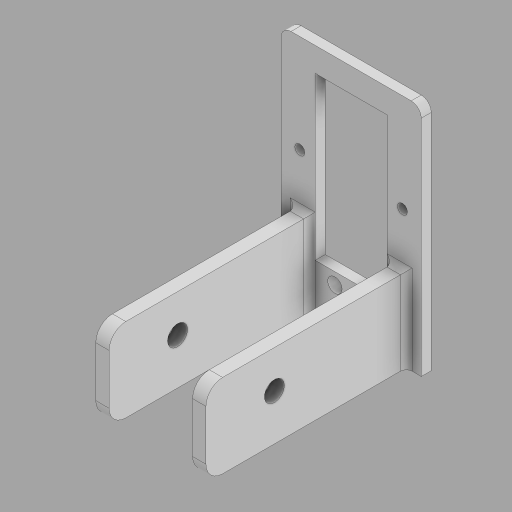
# Autodesk Inventor part: MG995_apoio
Saved by Autodesk Inventor 2023.2 (Build 272271030, 271C)
## iProperties
Created: 2023-04-15
Part Number: MG995_apoio
Material: Generic
Document SubType Name: Modeling
Designer: victo
Density: 1 g/cm^3
Appearance: Default
Author: victo
## iProperties of the stored document MG995_apoio_3DPrint.ipt
Created: 2023-07-24
Part Number: MG995_apoio_3DPrint
Material: Generic
Document SubType Name: Modeling
Designer: VICTOR
Density: 1 g/cm^3
Appearance: Default
Author: VICTOR
Autodesk Inventor part; units mm, degrees
ref_plane "YZ Plane" through (0, 0, 0) normal (1, 0, 0) x (0, 1, 0)
ref_plane "XZ Plane" through (0, 0, 0) normal (0, 1, 0) x (-1, 0, 0)
ref_plane "XY Plane" through (0, 0, 0) normal (0, 0, 1) x (1, 0, 0)
sketch "Sketch1" plane through (0, 0, 0) normal (0, 0, 1) x (1, 0, 0)
  line L0 (0, 0) -> (42, 0)
  line L1 (42, 0) -> (42, 70)
  line L2 (42, 70) -> (0, 70)
  line L3 (0, 70) -> (0, 0)
  line L4 (31.75, 14.25) -> (10.25, 14.25)
  line L5 (10.25, 14.25) -> (10.25, 55.75)
  line L6 (10.25, 55.75) -> (31.75, 55.75)
  line L7 (31.75, 55.75) -> (31.75, 14.25)
  line L8 (31.75, 14.25) -> (10.25, 55.75) construction
  line L9 (10.25, 14.25) -> (31.75, 55.75) construction
  line L10 (21, 70) -> (21, 0)
  line L11 (0, 35) -> (42, 35)
  point P0 (21, 35)
  point P1 (10.8, 7)
  point P2 (31.2, 7)
  point P3 (31.2, 0)
  point P4 (10.8, 0)
  point P5 (31.75, 35)
  point P6 (21, 35)
  point P7 (10.25, 35)
  point P8 (21, 14.25)
  point P9 (21, 55.75)
  dimension "d0" = 42
  dimension "d1" = 70
  dimension "d4" = 21.5
  dimension "d5" = 41.5
  constraints: 24 end point, 7 midpoint, 4 parallel, 2 horizontal, 2 perpendicular
  measures "d0" distance of L2.end L1.end
  measures "d1" distance of L1.end L0.end
  measures "d4" distance of L5.end L6.end
  measures "d5" distance of L4.end L5.end
extrude "Extrusion1" add sketch "Sketch1" along normal blind 2
fillet "Fillet3" radius 3 2 edges at (42, 70, 1) (0, 70, 1)
extrude "Extrusion11" cut sketch "Sketch1" along normal blind 6 contours L10 L11 L7 L4 | L4 L5 L11 L10 | L5 L6 L10 L11 | L10 L6 L7 L11
sketch "Sketch14" plane through (0, 0, 2) normal (0, 0, 1) x (1, 0, 0)
  line L0 (31.75, 55.75) -> (10.25, 55.75) projected
  circle A0 centre (16.15, 59.2) radius 2.15
  circle A1 centre (25.85, 59.2) radius 2.15
  line L1 (16.15, 59.2) -> (25.85, 59.2)
  line L2 (10.8, 35) -> (31.2, 35)
  circle A2 centre (16.15, 10.8) radius 2.15
  circle A3 centre (25.85, 10.8) radius 2.15
  line L3 (16.15, 10.8) -> (25.85, 10.8)
  line L4 (0, 0) -> (42, 0) projected
  arc A4 (3, 70) -> (0, 67) centre (3, 67) ccw projected
  line L5 (0, 67) -> (0, 0) projected
  line L6 (42, 0) -> (42, 67) projected
  arc A5 (42, 67) -> (39, 70) centre (39, 67) ccw projected
  line L7 (39, 70) -> (3, 70) projected
  point P0 (21, 59.2)
  dimension "d54" = 4.3
  dimension "d55" = 4.3
  dimension "d56" = 9.7
  constraints: 6 end point, 4 centre point, 2 symmetric about line, 1 horizontal, 1 midpoint, 2 other
  measures "d54" diameter of A0
  measures "d55" diameter of A1
  measures "d56" distance of L1.end L1.start
extrude "Extrusion12" cut sketch "Sketch14" against normal blind 6 contours A0 | A1 | A2 | A3
sketch "Sketch17" plane through (0, 0, 2) normal (0, 0, 1) x (1, 0, 0)
  circle A0 centre (16.15, 10.8) radius 2.15 projected
  circle A1 centre (25.85, 59.2) radius 2.15 projected
  circle A2 centre (25.85, 10.8) radius 2.15 projected
  circle A3 centre (16.15, 59.2) radius 2.15 projected
  line L0 (10.25, 55.75) -> (31.75, 55.75) projected
  line L1 (31.75, 55.75) -> (31.75, 14.25) projected
  line L2 (31.75, 14.25) -> (10.25, 14.25) projected
  line L3 (10.25, 14.25) -> (10.25, 55.75) projected
  circle A4 centre (16.15, 59.2) radius 2.15 projected
  circle A5 centre (25.85, 59.2) radius 2.15 projected
  line L4 (16.15, 61.35) -> (25.85, 61.35)
  line L5 (25.85, 59.2) -> (25.85, 61.35)
  line L6 (14, 59.2) -> (14, 55.75)
  line L7 (28, 59.2) -> (28, 55.75)
  line L8 (10.25, 55.75) -> (10.25, 14.25) projected
  line L9 (10.25, 55.75) -> (10.25, 62.75)
  line L10 (10.25, 62.75) -> (31.75, 62.75)
  line L11 (31.75, 62.75) -> (31.75, 55.75)
  line L12 (0, 0) -> (42, 0) projected
  arc A6 (3, 70) -> (0, 67) centre (3, 67) ccw projected
  line L13 (0, 67) -> (0, 0) projected
  line L14 (42, 0) -> (42, 67) projected
  arc A7 (42, 67) -> (39, 70) centre (39, 67) ccw projected
  line L15 (39, 70) -> (3, 70) projected
  dimension "d67" = 7
  constraints: 14 end point, 5 tangent, 4 perpendicular, 4 point on circle, 2 point on line, 2 vertical
  measures "d67" distance between parallel lines of L0 L10
extrude "Extrusion15" cut sketch "Sketch17" against normal blind 6 contours L7 L0 L6 A3 L4 A1 | A1 L4 A3 L6 L0 L9 L10 L11 L7
sketch "Sketch18" plane through (0, 0, 2) normal (0, 0, 1) x (1, 0, 0)
  line L0 (10.25, 14.25) -> (10.25, 62.75) projected
  line L1 (10.25, 62.75) -> (31.75, 62.75) projected
  line L2 (31.75, 62.75) -> (31.75, 14.25) projected
  line L3 (31.75, 14.25) -> (10.25, 14.25) projected
  circle A0 centre (25.85, 10.8) radius 2.15 projected
  circle A1 centre (16.15, 10.8) radius 2.15 projected
  line L4 (10.25, 40.625) -> (5.625, 40.625)
  line L5 (5.625, 40.625) -> (5.625, 69)
  circle A2 centre (5.625, 40.625) radius 1.5
  line L6 (21, 80.706) -> (21, -3.1342)
  circle A3 centre (36.375, 40.625) radius 1.5
  line L7 (0, 0) -> (42, 0) projected
  arc A4 (3, 70) -> (0, 67) centre (3, 67) ccw projected
  line L8 (0, 67) -> (0, 0) projected
  line L9 (42, 0) -> (42, 67) projected
  arc A5 (42, 67) -> (39, 70) centre (39, 67) ccw projected
  line L10 (39, 70) -> (3, 70) projected
  dimension "d70" = 4.625
  dimension "d71" = 28.375
  dimension "d72" = 3
  dimension "d75" = 30.75
  constraints: 6 end point, 2 centre point, 1 coincident, 1 horizontal, 1 point on line, 1 symmetric about line, 1 vertical, 1 other
  measures "d70" distance of L4.start L4.end
  measures "d71" distance of L4.end L5.end
  measures "d72" diameter of A2
  measures "d75" distance of A3.centre L4.end
extrude "Extrusion16" cut sketch "Sketch18" against normal blind 10 contours A2 L5 L4 | L4 L5 A2 | A3
sketch "Sketch22" plane through (0, 0, 2) normal (0, 0, 1) x (1, 0, 0)
  point P0 (0, 0)
sketch "Sketch23" plane through (0, 0, 2) normal (0, 0, 1) x (1, 0, 0)
  line L0 (0, 67) -> (0, 0) projected
  line L1 (0, 0) -> (0, 7)
  line L2 (0, 7) -> (42, 7)
  line L3 (42, 0) -> (42, 67) projected
  circle A0 centre (5.625, 40.625) radius 1.5 projected
  circle A1 centre (36.375, 40.625) radius 1.5 projected
  arc A2 (3, 70) -> (0, 67) centre (3, 67) ccw projected
  line L4 (0, 67) -> (0, 0) projected
  line L5 (0, 0) -> (42, 0) projected
  line L6 (42, 0) -> (42, 67) projected
  arc A3 (42, 67) -> (39, 70) centre (39, 67) ccw projected
  line L7 (39, 70) -> (3, 70) projected
  line L8 (10.25, 14.25) -> (10.25, 62.75) projected
  line L9 (10.25, 62.75) -> (31.75, 62.75) projected
  line L10 (31.75, 62.75) -> (31.75, 14.25) projected
  line L11 (31.75, 14.25) -> (10.25, 14.25) projected
  circle A4 centre (25.85, 10.8) radius 2.15 projected
  circle A5 centre (16.15, 10.8) radius 2.15 projected
  dimension "d88" = 7
  constraints: 4 end point, 2 point on line, 1 perpendicular
  measures "d88" distance of L0.end L1.end
extrude "Extrusion20" cut sketch "Sketch23" against normal blind 10 contours L2 L3 L5 L0
sketch "Sketch25" plane through (0, 0, 2) normal (0, 0, 1) x (1, 0, 0)
  line L0 (0, 67) -> (0, 7) projected
  line L1 (0, 7) -> (42, 7)
  line L2 (42, 7) -> (42, 0)
  line L3 (42, 0) -> (0, 0)
  line L4 (0, 0) -> (0, 7)
  dimension "d97" = 42
  dimension "d119" = 7
  constraints: 8 end point, 2 parallel, 1 horizontal, 1 perpendicular
  measures "d97" distance of L2.end L3.end
  measures "d119" distance of L3.end L0.end
extrude "Extrusion22" add sketch "Sketch25" along normal blind 60 and the other way blind 2
sketch "Sketch26" plane through (0, 0, 0) normal (-1, 0, 0) x (0, 0, 1)
  line L0 (2, 67) -> (2, 7) projected
  line L1 (0, 67) -> (2, 67) projected
  line L2 (0, 0) -> (62, 0) projected
  line L3 (62, 7) -> (62, 0) projected
  line L4 (62, 7) -> (2, 7) projected
  line L5 (2, 7) -> (4, 7) projected
  line L6 (2, 7) -> (22, 7)
  line L7 (4, 7) -> (47.3031, 7) projected
  line L8 (32.1962, 25) -> (62, 25)
  line L9 (2, 7) -> (62, 7) projected
  line L10 (62, 25) -> (62, 7)
  line L11 (32.1962, 25) -> (25.6515, 25)
  line L12 (0, 67) -> (0, 0) projected
  line L13 (22, 7) -> (22, 25)
  line L14 (25.6515, 25) -> (22, 25)
  dimension "d103" = 20
  dimension "d120" = 25
  constraints: 12 end point, 2 horizontal, 2 vertical, 1 perpendicular, 1 point on line
  measures "d103" distance of L0.end L6.end
  measures "d120" distance between parallel lines of L2 L8
extrude "Extrusion23" add sketch "Sketch26" against normal blind 42 contours L13 L14 L11 L8 L10 L4
sketch "Sketch27" plane through (0, 25, 62) normal (0, 1, 0) x (1, 0, 0)
  line L0 (0, 0) -> (0, 40) projected
  line L1 (0, 0) -> (42, 0) projected
  line L2 (42, 40) -> (42, 0) projected
  circle A0 centre (21, 19) radius 13
  line L3 (21, 19) -> (21, 0)
  line L4 (0, 0) -> (42, 0) projected
  line L5 (0, 40) -> (42, 40) projected
  point P0 (0, 62)
  dimension "d106" = 26
  dimension "d112" = 19
  constraints: 2 end point, 1 centre point, 1 midpoint
  measures "d106" diameter of A0
  measures "d112" distance of L3.start L3.end
extrude "Extrusion24" cut sketch "Sketch27" against normal blind 42 contours A0
sketch "Sketch30" plane through (0, 0, 0) normal (-1, 0, 0) x (0, 0, 1)
  point P0 (0, 0)
sketch "Sketch34" plane through (0, 0, 0) normal (0, 0, -1) x (-1, 0, 0)
  arc A0 (0, 67) -> (-3, 70) centre (-3, 67) ccw projected
  line L0 (-39, 70) -> (-3, 70) projected
  arc A1 (-39, 70) -> (-42, 67) centre (-39, 67) ccw projected
  line L1 (-42, 0) -> (-42, 67) projected
  line L2 (-42, 0) -> (0, 0) projected
  circle A2 centre (-25.85, 10.8) radius 2.15 projected
  circle A3 centre (-16.15, 10.8) radius 2.15 projected
  line L3 (-10.25, 62.75) -> (-10.25, 14.25) projected
  line L4 (-10.25, 14.25) -> (-31.75, 14.25) projected
  line L5 (-31.75, 14.25) -> (-31.75, 62.75) projected
  line L6 (-31.75, 62.75) -> (-10.25, 62.75) projected
  circle A4 centre (-36.375, 40.625) radius 1.5 projected
  circle A5 centre (-5.625, 40.625) radius 1.5 projected
  line L7 (0, 67) -> (0, 0) projected
extrude "Extrusion27" add sketch "Sketch34" along normal blind 1
sketch "Sketch36" plane through (0, 0, 62) normal (0, 0, 1) x (1, 0, 0)
  point P0 (0, 0)
sketch "Sketch37" plane through (0, 0, 62) normal (0, 0, 1) x (1, 0, 0)
  line L0 (34, 0) -> (8, 0) projected
  line L1 (8, 25) -> (34, 25) projected
  line L2 (8, 25) -> (34, 25) projected
  line L3 (0, 0) -> (8, 0)
  line L4 (8, 0) -> (8, 25)
  line L5 (8, 25) -> (0, 25)
  line L6 (0, 25) -> (0, 0)
  line L7 (42, 67) -> (42, 0) projected
  line L8 (42, 0) -> (34, 0)
  line L9 (34, 0) -> (34, 25)
  line L10 (34, 25) -> (42, 25)
  line L11 (42, 25) -> (42, 0)
  line L12 (0, 25) -> (42, 25) projected
  line L13 (4, 25) -> (4, 0)
  line L14 (42, 0) -> (0, 0) projected
  line L15 (38, 25) -> (38, 0)
  constraints: 20 end point, 4 parallel, 4 perpendicular, 3 point on line, 2 horizontal, 1 midpoint
extrude "Extrusion29" add sketch "Sketch37" against normal blind 60 contours L9 L10 L15 L8 | L3 L13 L5 L4
sketch "Sketch39" plane through (0, 25, 62) normal (0, 1, 0) x (1, 0, 0)
  circle A0 centre (21, 19) radius 13 projected
  line L0 (0, 0) -> (42, 0) projected
  line L1 (34, 60) -> (38, 60) projected
  line L2 (34, 40) -> (34, 60) projected
  line L3 (8, 40) -> (34, 40) projected
  line L4 (8, 40) -> (8, 60) projected
  line L5 (4, 60) -> (8, 60) projected
  line L6 (0, 0) -> (0, 40) projected
  line L7 (8, 0) -> (0, 0)
  line L8 (8, 40) -> (8, 0)
  line L9 (0, 0) -> (42, 0) projected
  line L10 (34, 40) -> (34, 0)
  line L11 (34, 40) -> (34, 60) projected
  line L12 (8, 60) -> (34, 60) projected
  line L13 (8, 60) -> (8, 40) projected
  line L14 (8, 40) -> (34, 40) projected
  line L15 (42, 40) -> (42, 0) projected
  line L16 (38, 40) -> (42, 40) projected
  line L17 (38, 40) -> (38, 60) projected
  line L18 (4, 40) -> (4, 60) projected
  line L19 (0, 40) -> (4, 40) projected
  point P0 (0, 62)
  point P1 (8, 19)
  point P2 (34, 19)
  constraints: 6 end point, 2 perpendicular, 2 point on line
extrude "Extrusion31" cut sketch "Sketch39" against normal blind 42 contours L10 L0 L8 A0 | A0 L8 L3 L10 | L3 L4 L12 L2
fillet "Fillet15" radius 5 6 edges at (6, 0, 62) (2, 0, 62) (2, 25, 62) (40, 25, 62) (40, 0, 62) (36, 0, 62)
extrude "Extrusion32" cut sketch "Sketch37" against normal blind 60 contours L15 L10 L7 L8 | L3 L6 L5 L13
sketch "Sketch40" plane through (8, 0, 2) normal (1, 0, 0) x (0, 0, -1)
  arc A0 (-55, 25) -> (-60, 20) centre (-55, 20) ccw projected
  line L0 (-60, 5) -> (-60, 20) projected
  arc A1 (-60, 5) -> (-55, 0) centre (-55, 5) ccw projected
  line L1 (0, 0) -> (-55, 0) projected
  line L2 (0, 25) -> (0, 0) projected
  line L3 (-55, 25) -> (0, 25) projected
  arc A2 (-55, 25) -> (-60, 20) centre (-55, 20) ccw projected
  line L4 (0, 25) -> (-55, 25) projected
  line L5 (0, 25) -> (0, 0) projected
  line L6 (-55, 0) -> (0, 0) projected
  arc A3 (-60, 5) -> (-55, 0) centre (-55, 5) ccw projected
  line L7 (-60, 20) -> (-60, 5) projected
  point P0 (2, 0)
extrude "Extrusion33" add sketch "Sketch40" along normal blind 0.5
sketch "Sketch41" plane through (34, 0, 2) normal (-1, 0, 0) x (0, 0, 1)
  arc A0 (60, 20) -> (55, 25) centre (55, 20) ccw projected
  line L0 (0, 25) -> (55, 25) projected
  line L1 (0, 25) -> (0, 0) projected
  line L2 (55, 0) -> (0, 0) projected
  arc A1 (55, 0) -> (60, 5) centre (55, 5) ccw projected
  line L3 (60, 20) -> (60, 5) projected
  point P0 (-2, 0)
extrude "Extrusion34" add sketch "Sketch41" along normal blind 0.5
sketch "Sketch42" plane through (4, 0, 2) normal (-1, 0, 0) x (0, 0, 1)
  line L0 (0, 25) -> (0, 0) projected
  line L1 (55, 0) -> (0, 0) projected
  arc A0 (55, 0) -> (60, 5) centre (55, 5) ccw projected
  line L2 (60, 20) -> (60, 5) projected
  arc A1 (60, 20) -> (55, 25) centre (55, 20) ccw projected
  line L3 (0, 25) -> (55, 25) projected
  point P0 (-2, 0)
extrude "Extrusion35" cut sketch "Sketch42" against normal blind 0.5
sketch "Sketch43" plane through (38, 0, 2) normal (1, 0, 0) x (0, 0, -1)
  line L0 (0, 0) -> (0, 25) projected
  line L1 (-55, 25) -> (0, 25) projected
  arc A0 (-55, 25) -> (-60, 20) centre (-55, 20) ccw projected
  line L2 (-60, 5) -> (-60, 20) projected
  arc A1 (-60, 5) -> (-55, 0) centre (-55, 5) ccw projected
  line L3 (0, 0) -> (-55, 0) projected
  point P0 (2, 0)
extrude "Extrusion36" cut sketch "Sketch43" against normal blind 0.5
fillet "Fillet18" radius 1.75 6 edges at (4.5, 12.5, 2) (6.5, 25, 2) (8.5, 12.5, 2) (33.5, 12.5, 2) (37.5, 12.5, 2) (35.5, 25, 2)
sketch "Sketch45" plane through (37.5, 0, 2) normal (1, 0, 0) x (0, 0, -1)
  line L0 (-1.75, 25) -> (-1.75, 0) projected
  line L1 (-55, 25) -> (-1.75, 25) projected
  arc A0 (-55, 25) -> (-60, 20) centre (-55, 20) ccw projected
  line L2 (-60, 5) -> (-60, 20) projected
  arc A1 (-60, 5) -> (-55, 0) centre (-55, 5) ccw projected
  line L3 (-1.75, 0) -> (-55, 0) projected
  line L4 (-60, 12.5) -> (-42.702, 12.5)
  line L5 (-39.5, 25) -> (-39.5, 13.711)
  circle A2 centre (-39.5, 13.711) radius 3
  point P0 (2, 0)
  dimension "d153" = 17.298
  dimension "d154" = 11.289
  dimension "d155" = 6
  dimension "d158" = 20.5
  constraints: 4 end point, 1 centre point, 1 coincident, 1 horizontal, 1 midpoint, 1 point on line, 1 vertical
  measures "d153" distance of L4.start L4.end
  measures "d154" distance of L5.start L5.end
  measures "d155" diameter of A2
  measures "d158" distance from line of L2 L5.end
extrude "Extrusion38" cut sketch "Sketch45" against normal blind 100 contours A2
body "Solid1"
